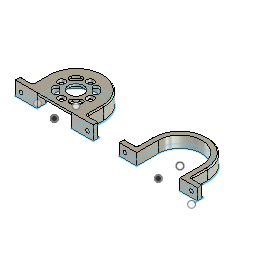
Крепеж Мотора550 v2 (Autodesk Fusion 360 design; units mm, degrees)
Autodesk Fusion 360 part; units mm, degrees
sketch "Sketch1" plane through (0, 0, 0) normal (0, 0, 1) x (1, 0, 0)
  line L0 (52.7317, 75.765) -> (52.7317, 80.765)
  line L1 (120.2317, 80.765) -> (120.2317, 75.765)
  line L2 (52.7317, 80.765) -> (62.7317, 80.765)
  line L3 (110.2317, 80.765) -> (120.2317, 80.765)
  line L4 (62.7317, 94.515) -> (62.7317, 80.765)
  line L5 (110.2317, 80.765) -> (110.2317, 94.515)
  arc A0 (110.2317, 94.515) -> (62.7317, 94.515) centre (86.4817, 94.515) ccw
  arc A1 (67.1168, 80.765) -> (67.7317, 79.9376) centre (86.4817, 94.515) ccw
  line L6 (195.2317, 75.765) -> (195.2317, 94.515)
  line L7 (210.2317, 80.765) -> (210.2317, 70.765)
  line L8 (200.2317, 80.765) -> (210.2317, 80.765)
  line L9 (200.2317, 80.765) -> (200.2317, 94.515)
  line L10 (142.7317, 80.765) -> (152.7317, 80.765)
  arc A2 (157.1168, 80.765) -> (157.7317, 79.9376) centre (176.4817, 94.515) ccw
  line L11 (152.7317, 94.515) -> (152.7317, 80.765)
  arc A3 (200.2317, 94.515) -> (152.7317, 94.515) centre (176.4817, 94.515) ccw
  line L12 (157.7317, 94.515) -> (157.7317, 75.765)
  line L13 (142.7317, 75.765) -> (142.7317, 80.765)
  line L14 (71.4817, 83.265) -> (71.4817, 75.765)
  line L15 (101.4817, 75.765) -> (101.4817, 83.265)
  arc A4 (101.4817, 83.265) -> (71.4817, 83.265) centre (86.4817, 94.515) ccw
  line L16 (52.7317, 75.765) -> (71.4817, 75.765)
  line L17 (101.4817, 75.765) -> (120.2317, 75.765)
  arc A5 (195.2317, 94.515) -> (157.7317, 94.515) centre (176.4817, 94.515) ccw
  line L18 (142.7317, 75.765) -> (157.7317, 75.765)
  line L19 (195.2317, 75.765) -> (210.2317, 75.765)
  point P0 (86.4817, 75.765)
  point P1 (86.4817, 75.765)
  point P2 (176.4817, 75.765)
  point P3 (176.4817, 75.765)
  point P4 (86.4817, 75.765)
  dimension "d1" = 37.5
  dimension "d3" = 47.5
  dimension "d4" = 67.5
  dimension "d6" = 37.5
  dimension "d7" = 47.5
  dimension "d8" = 67.5
  constraint parallel L0 L1
  constraint concentric A0 A4
  constraint coincident A1.start A0
  constraint collinear L2 L3
  constraint parallel L4 L5
  constraint tangent L5 A0
  constraint coincident P4 P1
  constraint concentric A0 A1
  constraint parallel L7 L13
  constraint midpoint L19.end L7
  constraint concentric A3 A5
  constraint coincident A2.start A3
  constraint collinear L8 L10
  constraint parallel L9 L11
  constraint tangent L9 A3
  constraint parallel L6 L12
  constraint coincident P3 P2
  constraint coincident L6.start L18
  constraint coincident A2.end L12
  constraint concentric A2 A3
  constraint parallel L14 L15
  constraint collinear L16 L17
  constraint collinear L18 L19
  measures "d1" diameter of A4
  measures "d3" diameter of A0
  measures "d4" distance of L0.end L1.start
  measures "d6" diameter of A5
  measures "d7" diameter of A3
  measures "d8" distance of L10.start L7.start
extrude "Extrude1" add sketch "Sketch1" along normal blind 10 contours L0 L1 L2 L3 L4 L5 A0 L14 L15 A4 L16 L17 makes body 1
extrude "Extrude2" add sketch "Sketch1" along normal blind 10 separate body contours L6 L7 L8 L9 L10 L11 A3 L12 L13 A5 L18 L19 makes body 2
hole "Hole1" at (205.2317, 80.765, 5) direction (0, -1, 0) diameter 3 depth 8 tip angle 118 bodies 2
hole "Hole2" at (147.7317, 80.765, 5) direction (0, -1, 0) diameter 3 depth 8 tip angle 118 bodies 2
hole "Hole3" at (115.2317, 80.765, 5) direction (0, -1, 0) diameter 3 depth 8 tip angle 118 bodies 1
hole "Hole4" at (57.7317, 80.765, 5) direction (0, -1, 0) diameter 3 depth 8 tip angle 118 bodies 1
sketch "Sketch2" plane through (0, 0, 10) normal (0, 0, 1) x (-1, 0, 0)
  line L0 (-101.4817, -83.265) -> (-101.4817, -75.765)
  line L1 (-101.4817, -75.765) -> (-120.2317, -75.765)
  line L2 (-120.2317, -75.765) -> (-120.2317, -80.765)
  line L3 (-120.2317, -80.765) -> (-110.2317, -80.765)
  line L4 (-110.2317, -80.765) -> (-110.2317, -94.515)
  arc A0 (-110.2317, -94.515) -> (-62.7317, -94.515) centre (-86.4817, -94.515) ccw
  line L5 (-62.7317, -94.515) -> (-62.7317, -80.765)
  line L6 (-62.7317, -80.765) -> (-52.7317, -80.765)
  line L7 (-52.7317, -80.765) -> (-52.7317, -75.765)
  line L8 (-52.7317, -75.765) -> (-71.4817, -75.765)
  line L9 (-71.4817, -75.765) -> (-71.4817, -83.265)
  arc A1 (-101.4817, -83.265) -> (-71.4817, -83.265) centre (-86.4817, -94.515) ccw
  line L10 (-71.4817, -75.765) -> (-101.4817, -75.765)
  circle A2 centre (-86.4817, -94.515) radius 6.65
  circle A3 centre (-98.9817, -94.515) radius 1.55
  circle A4 centre (-86.4817, -94.515) radius 12.5
  arc A5 (-78.1054, -106.9584) -> (-74.0383, -102.8913) centre (-86.4817, -94.515) ccw
  arc A6 (-80.8975, -102.8106) -> (-78.1054, -106.9584) centre (-79.5015, -104.8845) ccw
  arc A7 (-80.8975, -102.8106) -> (-78.1861, -100.0992) centre (-86.4817, -94.515) ccw
  arc A8 (-74.0383, -102.8913) -> (-78.1861, -100.0992) centre (-76.1122, -101.4952) ccw
  arc A9 (-79.5015, -104.8845) -> (-76.1122, -101.4952) centre (-86.4817, -94.515) ccw construction
  arc A10 (-74.0383, -86.1387) -> (-78.1054, -82.0716) centre (-86.4817, -94.515) ccw
  arc A11 (-78.1861, -88.9308) -> (-74.0383, -86.1387) centre (-76.1122, -87.5347) ccw
  arc A12 (-78.1861, -88.9308) -> (-80.8975, -86.2194) centre (-86.4817, -94.515) ccw
  arc A13 (-78.1054, -82.0716) -> (-80.8975, -86.2194) centre (-79.5015, -84.1455) ccw
  arc A14 (-94.858, -82.0716) -> (-98.9251, -86.1387) centre (-86.4817, -94.515) ccw
  arc A15 (-92.0659, -86.2194) -> (-94.858, -82.0716) centre (-93.462, -84.1455) ccw
  arc A16 (-92.0659, -86.2194) -> (-94.7773, -88.9308) centre (-86.4817, -94.515) ccw
  arc A17 (-98.9251, -86.1387) -> (-94.7773, -88.9308) centre (-96.8512, -87.5347) ccw
  arc A18 (-98.9251, -102.8913) -> (-94.858, -106.9584) centre (-86.4817, -94.515) ccw
  arc A19 (-94.7773, -100.0992) -> (-98.9251, -102.8913) centre (-96.8512, -101.4952) ccw
  arc A20 (-94.7773, -100.0992) -> (-92.0659, -102.8106) centre (-86.4817, -94.515) ccw
  arc A21 (-94.858, -106.9584) -> (-92.0659, -102.8106) centre (-93.462, -104.8845) ccw
  arc A22 (-101.0591, -75.765) -> (-71.9043, -75.765) centre (-86.4817, -94.515) ccw
  circle A23 centre (-86.4817, -107.015) radius 1.55
  circle A24 centre (-73.9817, -94.515) radius 1.55
  circle A25 centre (-86.4817, -82.015) radius 1.55
  point P0 (-77.6281, -103.339)
  dimension "d26" = 13.3
  dimension "d28" = 3.1
  dimension "d29" = 12.5
  dimension "d32" = 12.5
  dimension "d33" = 5
  dimension "d34" = 2.3869
  dimension "d35" = 4.7931
  dimension "d37" = 360
  dimension "d44" = 360
  constraint concentric A0 A22
  constraint coincident L8.end L9.start
  constraint coincident L0.end L1.start
  constraint concentric A2 A22
  constraint concentric A2 A4
  constraint coincident P0 A4
  constraint tangent A5 A6
  constraint tangent A6 A7
  constraint tangent A7 A8
  constraint tangent A5 A8
  constraint coincident A4 A6.centre
  constraint coincident A4 A8.centre
  constraint coincident L10 A22.end
  constraint coincident L10 A22.start
  measures "d26" diameter of A2
  measures "d28" diameter of A3
  measures "d29" distance of A0.centre A3.centre
  measures "d32" distance of A0.centre P0
  measures "d33" diameter of A8
  measures "d34" distance of P0 A8.centre
  measures "d35" distance of A8.centre A6.centre
extrude "Extrude3" add sketch "Sketch2" along normal blind 2 separate body contours L0 L9 A1 L10 A22 | A3 A4 A6 A7 A8 A11 A12 A13 A15 A16 A17 A19 A20 A21 A23 A24 A25 makes body 3
extrude "Extrude4" add 1 faces at (104.3984, 79.9316, 10) along direction (0, 0, 1) blind 2 on bodies 1 bodies 1 3
chamfer "Chamfer2" distance 1.5 angle 45 4 edges at (87.9268, 106.4545, 12) (75.4268, 93.9545, 12) (87.9268, 81.4545, 12) (100.4268, 93.9545, 12) on bodies 1
chamfer "Chamfer3" distance 2 angle 45 4 edges at (115.7741, 80.765, 3.6015) (58.2741, 80.765, 3.6015) (205.7741, 80.765, 3.6015) (148.2741, 80.765, 3.6015) on bodies 1 2
fillet "Fillet2" radius 1 5 faces at (179.4349, 118.0807, 6.6667) (152.7317, 89.9316, 3.3333) (200.2317, 85.3483, 3.3333) (143.235, 80.765, 4.9128) (200.735, 80.765, 5.0872) on bodies 2
fillet "Fillet3" radius 1 5 faces at (108.3668, 103.7403, 8) (62.7317, 89.9316, 4) (110.2317, 85.3483, 4) (57.7317, 80.765, 10.8333) (115.2317, 80.765, 10.8333) on bodies 1
named bodies: "КрепежМотораПеред", "КрепежМотора2"
